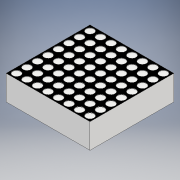
# Autodesk Inventor part: DISP LED 8x8 1.9 DIP-16
Saved by Autodesk Inventor 2017 (Build 210142000, 142)
## iProperties
Created: 2017-10-17
Part Number: DISP LED 8x8 1.9 DIP-16
Material: Generic
Document SubType Name: Modeling
Designer: danil
Density: 1 g/cm^3
Appearance: Default
Author: danil
Autodesk Inventor part; units mm, degrees
ref_plane "YZ Plane" through (0, 0, 0) normal (1, 0, 0) x (0, 1, 0)
ref_plane "XZ Plane" through (0, 0, 0) normal (0, 1, 0) x (-1, 0, 0)
ref_plane "XY Plane" through (0, 0, 0) normal (0, 0, 1) x (1, 0, 0)
sketch "Sketch1" plane through (0, 0, 0) normal (0, 0, 1) x (1, 0, 0)
  line L0 (-10, -10) -> (10, -10)
  line L1 (10, -10) -> (10, 10)
  line L2 (10, 10) -> (-10, 10)
  line L3 (-10, 10) -> (-10, -10)
  line L4 (-10, -10) -> (10, 10) construction
  line L5 (10, -10) -> (-10, 10) construction
  point P0 (0, 0)
  dimension "d0" = 20
  dimension "d1" = 20
  constraints: 12 end point, 2 midpoint, 2 parallel, 1 horizontal, 1 perpendicular
  measures "d0" distance of L2.end L1.end
  measures "d1" distance of L1.end L0.end
extrude "Extrusion1" add sketch "Sketch1" along normal blind 5.9
sketch "Sketch5" plane through (0, 0, 0) normal (0, 0, -1) x (-1, 0, 0)
  line L0 (10, -10) -> (-10, -10) projected
  line L1 (10, 10) -> (10, -10) projected
  line L2 (-10, 10) -> (10, 10) projected
  line L3 (-10, -10) -> (-10, 10) projected
  line L4 (-9.7, 9.7) -> (9.7, 9.7)
  line L5 (9.7, 9.7) -> (9.7, -9.7)
  line L6 (9.7, -9.7) -> (-9.7, -9.7)
  line L7 (-9.7, -9.7) -> (-9.7, 9.7)
  point P0 (0, 0)
  dimension "d28" = 0.3
  constraints: 8 end point, 3 other
  measures "d28" distance between parallel lines of L3 L7
extrude "Extrusion6" cut sketch "Sketch5" against normal blind 0.5 contours L4 L5 L6 L7
sketch "Sketch2" plane through (0, 0, 0.5) normal (0, 0, -1) x (-1, 0, 0)
  circle A0 centre (-8.75, -7.5) radius 0.255
  line L0 (-10, -10) -> (-10, 10)
  line L1 (10, -10) -> (-10, -10)
  circle A1 centre (-8.75, 7.5) radius 0.255
  circle A2 centre (-6.25, -7.5) radius 0.255
  circle A3 centre (-6.25, 7.5) radius 0.255
  circle A4 centre (-3.75, -7.5) radius 0.255
  circle A5 centre (-3.75, 7.5) radius 0.255
  circle A6 centre (-1.25, -7.5) radius 0.255
  circle A7 centre (-1.25, 7.5) radius 0.255
  circle A8 centre (1.25, -7.5) radius 0.255
  circle A9 centre (1.25, 7.5) radius 0.255
  circle A10 centre (3.75, -7.5) radius 0.255
  circle A11 centre (3.75, 7.5) radius 0.255
  circle A12 centre (6.25, -7.5) radius 0.255
  circle A13 centre (6.25, 7.5) radius 0.255
  circle A14 centre (8.75, -7.5) radius 0.255
  circle A15 centre (8.75, 7.5) radius 0.255
  line L2 (-1.25, 7.5) -> (1.25, 7.5)
  line L3 (0, 7.5) -> (0, -7.5)
  line L4 (-1.25, -7.5) -> (1.25, -7.5)
  point P0 (0, 0)
  point P1 (0, 0)
  dimension "d4" = 0.51
  dimension "d7" = 15
  dimension "d10" = 2.5
  constraints: 16 centre point, 10 end point, 3 midpoint, 2 horizontal, 2 vertical, 1 coincident, 1 parallel, 30 other
  measures "d4" diameter of A0
  measures "d7" distance of A0.centre A1.centre
  measures "d10" distance of A0.centre A2.centre
extrude "Extrusion2" add sketch "Sketch2" along normal blind 1.5
fillet "Fillet1" radius 0.15 16 edges at (1.505, -7.5, -1) (-0.995, -7.5, -1) (-3.495, -7.5, -1) (-5.995, -7.5, -1) (-8.495, -7.5, -1) (4.005, -7.5, -1) (6.505, -7.5, -1) (9.005, -7.5, -1) (9.005, 7.5, -1) (6.505, 7.5, -1) (4.005, 7.5, -1) (1.505, 7.5, -1) (-0.995, 7.5, -1) (-3.495, 7.5, -1) (-5.995, 7.5, -1) (-8.495, 7.5, -1)
sketch "Sketch3" plane through (0, 0, 5.9) normal (0, 0, 1) x (1, 0, 0)
  circle A0 centre (-8.75, -8.75) radius 0.95
  line L0 (-10, 10) -> (-10, -10) projected
  line L1 (-10, -10) -> (10, -10) projected
  circle A1 centre (-8.75, -6.25) radius 0.95
  circle A2 centre (-8.75, -3.75) radius 0.95
  circle A3 centre (-8.75, -1.25) radius 0.95
  circle A4 centre (-8.75, 1.25) radius 0.95
  circle A5 centre (-8.75, 3.75) radius 0.95
  circle A6 centre (-8.75, 6.25) radius 0.95
  circle A7 centre (-8.75, 8.75) radius 0.95
  circle A8 centre (-6.25, -8.75) radius 0.95
  circle A9 centre (-6.25, -6.25) radius 0.95
  circle A10 centre (-6.25, -3.75) radius 0.95
  circle A11 centre (-6.25, -1.25) radius 0.95
  circle A12 centre (-6.25, 1.25) radius 0.95
  circle A13 centre (-6.25, 3.75) radius 0.95
  circle A14 centre (-6.25, 6.25) radius 0.95
  circle A15 centre (-6.25, 8.75) radius 0.95
  circle A16 centre (-3.75, -8.75) radius 0.95
  circle A17 centre (-3.75, -6.25) radius 0.95
  circle A18 centre (-3.75, -3.75) radius 0.95
  circle A19 centre (-3.75, -1.25) radius 0.95
  circle A20 centre (-3.75, 1.25) radius 0.95
  circle A21 centre (-3.75, 3.75) radius 0.95
  circle A22 centre (-3.75, 6.25) radius 0.95
  circle A23 centre (-3.75, 8.75) radius 0.95
  circle A24 centre (-1.25, -8.75) radius 0.95
  circle A25 centre (-1.25, -6.25) radius 0.95
  circle A26 centre (-1.25, -3.75) radius 0.95
  circle A27 centre (-1.25, -1.25) radius 0.95
  circle A28 centre (-1.25, 1.25) radius 0.95
  circle A29 centre (-1.25, 3.75) radius 0.95
  circle A30 centre (-1.25, 6.25) radius 0.95
  circle A31 centre (-1.25, 8.75) radius 0.95
  circle A32 centre (1.25, -8.75) radius 0.95
  circle A33 centre (1.25, -6.25) radius 0.95
  circle A34 centre (1.25, -3.75) radius 0.95
  circle A35 centre (1.25, -1.25) radius 0.95
  circle A36 centre (1.25, 1.25) radius 0.95
  circle A37 centre (1.25, 3.75) radius 0.95
  circle A38 centre (1.25, 6.25) radius 0.95
  circle A39 centre (1.25, 8.75) radius 0.95
  circle A40 centre (3.75, -8.75) radius 0.95
  circle A41 centre (3.75, -6.25) radius 0.95
  circle A42 centre (3.75, -3.75) radius 0.95
  circle A43 centre (3.75, -1.25) radius 0.95
  circle A44 centre (3.75, 1.25) radius 0.95
  circle A45 centre (3.75, 3.75) radius 0.95
  circle A46 centre (3.75, 6.25) radius 0.95
  circle A47 centre (3.75, 8.75) radius 0.95
  circle A48 centre (6.25, -8.75) radius 0.95
  circle A49 centre (6.25, -6.25) radius 0.95
  circle A50 centre (6.25, -3.75) radius 0.95
  circle A51 centre (6.25, -1.25) radius 0.95
  circle A52 centre (6.25, 1.25) radius 0.95
  circle A53 centre (6.25, 3.75) radius 0.95
  circle A54 centre (6.25, 6.25) radius 0.95
  circle A55 centre (6.25, 8.75) radius 0.95
  circle A56 centre (8.75, -8.75) radius 0.95
  circle A57 centre (8.75, -6.25) radius 0.95
  circle A58 centre (8.75, -3.75) radius 0.95
  circle A59 centre (8.75, -1.25) radius 0.95
  circle A60 centre (8.75, 1.25) radius 0.95
  circle A61 centre (8.75, 3.75) radius 0.95
  circle A62 centre (8.75, 6.25) radius 0.95
  circle A63 centre (8.75, 8.75) radius 0.95
  line L2 (-1.25, 1.25) -> (1.25, -1.25)
  line L3 (-1.25, -1.25) -> (1.25, 1.25)
  point P0 (0, 0)
  point P1 (0, 0)
  dimension "d15" = 1.9
  dimension "d18" = 2.5
  dimension "d21" = 2.5
  constraints: 64 centre point, 4 end point, 2 coincident, 1 horizontal, 1 midpoint, 1 vertical, 126 other
  measures "d15" diameter of A0
  measures "d18" distance of A0.centre A1.centre
  measures "d21" distance of A0.centre A8.centre
extrude "Extrusion3" cut sketch "Sketch3" against normal blind 0.1
sketch "Sketch4" plane through (0, 0, 5.9) normal (0, 0, 1) x (1, 0, 0)
  circle A0 centre (8.75, 6.25) radius 0.95 projected
  circle A1 centre (8.75, 1.25) radius 0.95 projected
  circle A2 centre (8.75, -3.75) radius 0.95 projected
  circle A3 centre (8.75, -8.75) radius 0.95 projected
  circle A4 centre (6.25, 6.25) radius 0.95 projected
  circle A5 centre (6.25, 1.25) radius 0.95 projected
  circle A6 centre (6.25, -3.75) radius 0.95 projected
  circle A7 centre (6.25, -8.75) radius 0.95 projected
  circle A8 centre (3.75, 6.25) radius 0.95 projected
  circle A9 centre (3.75, 1.25) radius 0.95 projected
  circle A10 centre (3.75, -3.75) radius 0.95 projected
  circle A11 centre (3.75, -8.75) radius 0.95 projected
  circle A12 centre (1.25, 6.25) radius 0.95 projected
  circle A13 centre (1.25, 1.25) radius 0.95 projected
  circle A14 centre (1.25, -3.75) radius 0.95 projected
  circle A15 centre (1.25, -8.75) radius 0.95 projected
  circle A16 centre (-1.25, 6.25) radius 0.95 projected
  circle A17 centre (-1.25, 1.25) radius 0.95 projected
  circle A18 centre (-1.25, -3.75) radius 0.95 projected
  circle A19 centre (-1.25, -8.75) radius 0.95 projected
  circle A20 centre (-3.75, 6.25) radius 0.95 projected
  circle A21 centre (-3.75, 1.25) radius 0.95 projected
  circle A22 centre (-3.75, -3.75) radius 0.95 projected
  circle A23 centre (-3.75, -8.75) radius 0.95 projected
  circle A24 centre (-6.25, 6.25) radius 0.95 projected
  circle A25 centre (-6.25, 1.25) radius 0.95 projected
  circle A26 centre (-6.25, -3.75) radius 0.95 projected
  circle A27 centre (-6.25, -8.75) radius 0.95 projected
  circle A28 centre (-8.75, 6.25) radius 0.95 projected
  circle A29 centre (-8.75, 1.25) radius 0.95 projected
  circle A30 centre (-8.75, -3.75) radius 0.95 projected
  circle A31 centre (-8.75, -8.75) radius 0.95 projected
  circle A32 centre (-8.75, -6.25) radius 0.95 projected
  circle A33 centre (-8.75, -1.25) radius 0.95 projected
  circle A34 centre (-8.75, 3.75) radius 0.95 projected
  circle A35 centre (-8.75, 8.75) radius 0.95 projected
  circle A36 centre (-6.25, -6.25) radius 0.95 projected
  circle A37 centre (-6.25, -1.25) radius 0.95 projected
  circle A38 centre (-6.25, 3.75) radius 0.95 projected
  circle A39 centre (-6.25, 8.75) radius 0.95 projected
  circle A40 centre (-3.75, -6.25) radius 0.95 projected
  circle A41 centre (-3.75, -1.25) radius 0.95 projected
  circle A42 centre (-3.75, 3.75) radius 0.95 projected
  circle A43 centre (-3.75, 8.75) radius 0.95 projected
  circle A44 centre (-1.25, -6.25) radius 0.95 projected
  circle A45 centre (-1.25, -1.25) radius 0.95 projected
  circle A46 centre (-1.25, 3.75) radius 0.95 projected
  circle A47 centre (-1.25, 8.75) radius 0.95 projected
  circle A48 centre (1.25, -6.25) radius 0.95 projected
  circle A49 centre (1.25, -1.25) radius 0.95 projected
  circle A50 centre (1.25, 3.75) radius 0.95 projected
  circle A51 centre (1.25, 8.75) radius 0.95 projected
  circle A52 centre (3.75, -6.25) radius 0.95 projected
  circle A53 centre (3.75, -1.25) radius 0.95 projected
  circle A54 centre (3.75, 3.75) radius 0.95 projected
  circle A55 centre (3.75, 8.75) radius 0.95 projected
  circle A56 centre (6.25, -6.25) radius 0.95 projected
  circle A57 centre (6.25, -1.25) radius 0.95 projected
  circle A58 centre (6.25, 3.75) radius 0.95 projected
  circle A59 centre (6.25, 8.75) radius 0.95 projected
  circle A60 centre (8.75, -6.25) radius 0.95 projected
  circle A61 centre (8.75, -1.25) radius 0.95 projected
  circle A62 centre (8.75, 3.75) radius 0.95 projected
  circle A63 centre (8.75, 8.75) radius 0.95 projected
  line L0 (-10, -10) -> (10, -10) projected
  line L1 (10, -10) -> (10, 10) projected
  line L2 (10, 10) -> (-10, 10) projected
  line L3 (-10, 10) -> (-10, -10) projected
  point P0 (0, 0)
extrude "Extrusion4" add sketch "Sketch4" along normal blind 0.001
body "Solid1"
